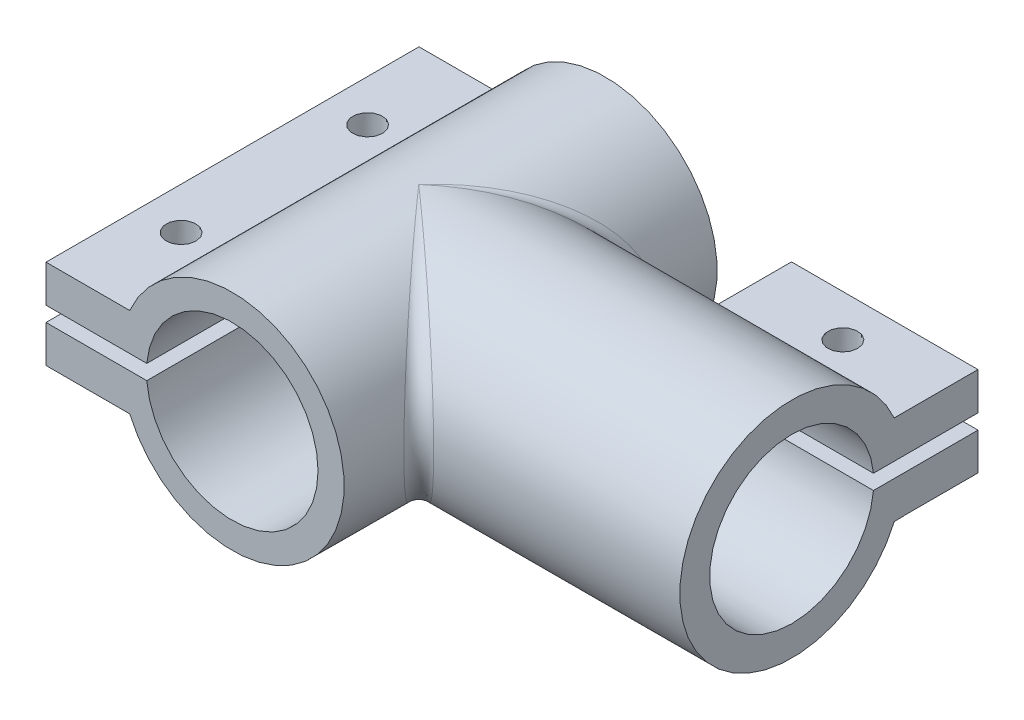
# Autodesk Inventor part: Tconection
Saved by Autodesk Inventor 2023 (Build 270158000, 158)
## iProperties
Created: 2023-09-25
Part Number: Tconection
Material: Generic
Document SubType Name: Modeling
Designer: Nikita
Density: 1 g/cm^3
Appearance: Default
Author: Nikita
Autodesk Inventor part; units mm, degrees
ref_plane "YZ Plane" through (0, 0, 0) normal (1, 0, 0) x (0, 1, 0)
ref_plane "XZ Plane" through (0, 0, 0) normal (0, 1, 0) x (-1, 0, 0)
ref_plane "XY Plane" through (0, 0, 0) normal (0, 0, 1) x (1, 0, 0)
sketch "Sketch1" plane through (0, 0, 0) normal (0, 0, 1) x (1, 0, 0)
  circle A0 centre (0, 0) radius 11.5
  circle A1 centre (0, 0) radius 15
  dimension "d0" = 23
  dimension "d1" = 30
  constraints: 2 centre point, 2 coincident
  measures "d0" diameter of A0
  measures "d1" diameter of A1
extrude "Extrusion1" add sketch "Sketch1" along normal blind 50
sketch "Sketch2" plane through (0, 0, 0) normal (0, 1, 0) x (-1, 0, 0)
  line L0 (0, 0) -> (0, 25) construction
  line L1 (0, 25) -> (-50, 25) construction
  dimension "d4" = 25
  dimension "d5" = 50
  constraints: 4 end point, 1 horizontal, 1 vertical
  measures "d4" distance of L0.start L0.end
  measures "d5" distance of L0.end L1.end
ref_plane "Work Plane1" through (50, 0, 25) normal (1, 0, 0) x (0, 1, 0)
sketch "Sketch3" plane through (50, 0, 25) normal (1, 0, 0) x (0, 1, 0)
  circle A0 centre (0, 0) radius 15
  point P0 (0, -25)
  dimension "d7" = 30
  constraints: 1 centre point
  measures "d7" diameter of A0
extrude "Extrusion2" add sketch "Sketch3" against normal up to next
sketch "Sketch4" plane through (50, 0, 25) normal (1, 0, 0) x (0, 0, -1)
  circle A0 centre (0, 0) radius 11
  point P0 (25, 0)
  dimension "d10" = 22
  constraints: 1 centre point
  measures "d10" diameter of A0
extrude "Extrusion3" cut sketch "Sketch4" against normal blind 48.5
fillet "Fillet1" radius 2 2 edges at (10.6066, -10.6066, 35.6066) (10.6066, 10.6066, 35.6066)
fillet "Fillet2" radius 2 2 edges at (10.6066, -10.6066, 14.3934) (10.6066, 10.6066, 14.3934)
sketch "Sketch5" plane through (0, 0, 0) normal (0, 0, -1) x (-1, 0, 0)
  circle A0 centre (0, 0) radius 11.5 projected
  line L0 (11.5, -1) -> (15.0466, -1)
  line L1 (15.0466, -1) -> (15.0466, 1)
  line L2 (15.0466, 1) -> (11.3539, 1)
  line L3 (11.3539, 1) -> (11.3539, -1)
  line L4 (11.3539, -1) -> (11.5, -1)
  constraints: 10 end point, 4 perpendicular, 1 point on line
extrude "Extrusion4" cut sketch "Sketch5" against normal blind 63 contours A0 L4 L3 L2 | A0 L2 L1 L0 L4 picked at (11.401, -0.1112)
sketch "Sketch6" plane through (0, 0, 0) normal (0, 0, -1) x (-1, 0, 0)
  arc A0 (14.9666, 1) -> (14.9666, -1) centre (0, 0) ccw projected
  line L0 (14.9666, 1) -> (14.9666, 6)
  line L1 (14.9666, 6) -> (13.7477, 6)
  dimension "d19" = 5
  constraints: 4 end point, 1 perpendicular, 1 point on circle, 1 vertical
  measures "d19" distance of L0.start L0.end
extrude "Extrusion5" add sketch "Sketch6" against normal blind 50
sketch "Sketch7" plane through (0, 0, 0) normal (0, 0, -1) x (-1, 0, 0)
  arc A0 (13.7477, 6) -> (14.9666, -1) centre (0, 0) ccw projected
  line L0 (14.9666, -1) -> (14.9666, -6)
  line L1 (14.9666, -6) -> (13.7477, -6)
  dimension "d22" = 5
  constraints: 4 end point, 1 perpendicular, 1 point on circle, 1 vertical
  measures "d22" distance of L0.start L0.end
extrude "Extrusion6" add sketch "Sketch7" against normal blind 50
sketch "Sketch8" plane through (-14.9666, 1, 0) normal (-1, 0, 0) x (0, 0, 1)
  line L0 (0, 5) -> (50, 5) projected
  line L1 (0, 0) -> (50, 0) projected
  line L2 (0, 5) -> (50, 5)
  line L3 (50, 5) -> (50, 0)
  line L4 (50, 0) -> (0, 0)
  line L5 (0, 0) -> (0, 5)
  point P0 (0, -1)
  constraints: 8 end point, 2 parallel, 1 horizontal, 1 perpendicular
extrude "Extrusion7" add sketch "Sketch8" along normal blind 10
sketch "Sketch9" plane through (-14.9666, -6, 0) normal (-1, 0, 0) x (0, 0, 1)
  line L0 (50, 0) -> (0, 0) projected
  line L1 (0, 5) -> (50, 5)
  line L2 (50, 5) -> (50, 0)
  line L3 (50, 0) -> (0, 0)
  line L4 (0, 0) -> (0, 5)
  point P0 (0, 6)
  constraints: 8 end point, 2 parallel, 1 horizontal, 1 perpendicular
extrude "Extrusion8" add sketch "Sketch9" along normal blind 10
sketch "Sketch10" plane through (-13.7477, 6, 50) normal (0, 1, 0) x (1, 0, 0)
  line L0 (-11.2189, 50) -> (2.2913, 50) construction
  line L1 (-11.2189, 50) -> (-11.2189, 25) construction
  line L2 (-11.2189, 0) -> (-11.2189, 50) construction
  line L3 (0, 50) -> (28.7477, 50) construction
  line L4 (-11.2189, 25) -> (0, 50) construction
  line L5 (0, 50) -> (-11.2189, 50) construction
  line L6 (-11.2189, 50) -> (0, 25) construction
  line L7 (0, 0) -> (0, 50) construction
  circle A0 centre (-5.6095, 37.5) radius 2
  point P0 (13.7477, 50)
  dimension "d29" = 25
  dimension "d30" = 4
  constraints: 8 end point, 3 midpoint, 1 centre point, 1 perpendicular
  measures "d29" distance of L0.start L1.end
  measures "d30" diameter of A0
extrude "Extrusion9" cut sketch "Sketch10" against normal blind 25.75
sketch "Sketch11" plane through (-13.7477, 6, 50) normal (0, 1, 0) x (1, 0, 0)
  line L0 (-11.2189, 50) -> (-11.2189, 0) construction
  line L1 (-11.2189, 0) -> (-11.2189, 25) construction
  line L2 (-11.2189, 25) -> (0, 25) construction
  line L3 (0, 0) -> (0, 50) construction
  line L4 (-11.2189, 0) -> (-0.3348, 25) construction
  line L5 (0, 0) -> (-11.2189, 0) construction
  line L6 (-11.2189, 25) -> (0, 0) construction
  circle A0 centre (-5.6095, 12.5) radius 2
  point P0 (13.7477, 50)
  dimension "d33" = 25
  dimension "d34" = 4
  constraints: 8 end point, 3 midpoint, 1 centre point, 1 point on line
  measures "d33" distance of L0.end L1.end
  measures "d34" diameter of A0
extrude "Extrusion10" cut sketch "Sketch11" against normal blind 25.75
sketch "Sketch12" plane through (50, 0, 25) normal (1, 0, 0) x (0, 0, -1)
  line L0 (12.133, 1) -> (15.2784, 1)
  line L1 (-25, 1) -> (25, 1) projected
  line L2 (15.2784, 1) -> (15.2784, -1)
  line L3 (15.2784, -1) -> (10.7779, -1)
  line L4 (10.7779, -1) -> (10.7779, 1)
  line L5 (10.7779, 1) -> (12.133, 1)
  point P0 (25, 0)
  dimension "d38" = 2
  constraints: 10 end point, 4 perpendicular, 2 point on line
  measures "d38" distance of L0.end L2.end
extrude "Extrusion11" cut sketch "Sketch12" against normal blind 25
sketch "Sketch13" plane through (50, 0, 25) normal (1, 0, 0) x (0, 0, -1)
  arc A0 (0, -15) -> (0, 15) centre (0, 0) ccw projected
  line L0 (14.9642, 1.036) -> (14.9642, 6.036)
  line L1 (14.9642, 6.036) -> (13.7319, 6.036)
  line L2 (10.9545, 1) -> (14.9666, 1) projected
  arc A1 (14.9666, 1) -> (13.7319, 6.036) centre (0, 0) ccw
  point P0 (25, 0)
  dimension "d41" = 5
  constraints: 4 end point, 4 point on circle, 1 centre point, 1 concentric, 1 perpendicular, 1 vertical
  measures "d41" distance of L0.start L0.end
extrude "Extrusion12" add sketch "Sketch13" against normal blind 25
sketch "Sketch14" plane through (50, 0, 25) normal (1, 0, 0) x (0, 0, -1)
  line L0 (14.9666, -1) -> (10.9545, -1) projected
  line L1 (14.9666, -1) -> (14.9666, -6)
  line L2 (14.9666, -6) -> (13.7606, -6)
  line L3 (13.7606, -6) -> (13.7606, -1)
  line L4 (14.9666, -1) -> (13.7606, -1)
  point P0 (25, 0)
  dimension "d44" = 5
  constraints: 8 end point, 2 perpendicular, 1 horizontal, 1 point on line, 1 vertical
  measures "d44" distance of L0.start L1.end
extrude "Extrusion13" add sketch "Sketch14" against normal blind 25
sketch "Sketch15" plane through (50, 1.036, 10.0358) normal (0, 0, -1) x (-1, 0, 0)
  line L0 (25, -0.036) -> (25, -2.036) projected
  line L1 (0, 5) -> (25, 5)
  line L2 (25, 5) -> (25, -0.036)
  line L3 (25, -0.036) -> (0, -0.036)
  line L4 (0, -0.036) -> (0, 5)
  point P0 (50, -1.036)
  constraints: 8 end point, 2 parallel, 1 coincident, 1 horizontal, 1 perpendicular
extrude "Extrusion14" add sketch "Sketch15" along normal blind 10
sketch "Sketch16" plane through (50, -6, 10.0334) normal (0, 0, -1) x (-1, 0, 0)
  line L0 (25, 0.0296) -> (25, 5) projected
  line L1 (0, 5) -> (25, 5)
  line L2 (25, 5) -> (25, 0.0296)
  line L3 (25, 0.0296) -> (0, 0.0296)
  line L4 (0, 0.0296) -> (0, 5)
  point P0 (50, 6)
  constraints: 8 end point, 2 parallel, 1 horizontal, 1 perpendicular
extrude "Extrusion15" add sketch "Sketch16" along normal blind 10
sketch "Sketch17" plane through (25, 6.036, 11.2681) normal (0, 1, 0) x (1, 0, 0)
  line L0 (25, 0.226) -> (0, 11.2681) construction
  line L1 (25, -2.7775) -> (25, 11.2322) construction
  line L2 (25, 11.2322) -> (0, 0) construction
  circle A0 centre (12.5, 5.6161) radius 2
  point P0 (-25, 11.2681)
  dimension "d51" = 4
  constraints: 4 end point, 1 centre point, 1 midpoint
  measures "d51" diameter of A0
extrude "Extrusion16" cut sketch "Sketch17" against normal blind 18.5
body "Solid1"
